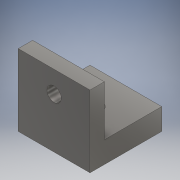
# Autodesk Inventor part: supportPoulie
Saved by Autodesk Inventor 2017 (Build 210142000, 142)
## iProperties
Created: 2017-10-26
Part Number: supportPoulie
Material: Stainless Steel
Document SubType Name: Modeling
Designer: Biscuit
Density: 8 g/cm^3
Appearance: Semi-Polished
Author: Biscuit
Autodesk Inventor part; units mm, degrees
ref_plane "YZ Plane" through (0, 0, 0) normal (1, 0, 0) x (0, 1, 0)
ref_plane "XZ Plane" through (0, 0, 0) normal (0, 1, 0) x (-1, 0, 0)
ref_plane "XY Plane" through (0, 0, 0) normal (0, 0, 1) x (1, 0, 0)
sketch "Sketch1" plane through (0, 0, 0) normal (0, 0, 1) x (1, 0, 0)
  line L0 (0, 0) -> (10, 0)
  line L1 (10, 0) -> (10, 10)
  line L2 (10, 10) -> (0, 10)
  line L3 (0, 10) -> (0, 0)
  circle A0 centre (5, 5) radius 1.5
  dimension "d0" = 10
  dimension "d1" = 10
  dimension "d8" = 3
  constraints: 8 end point, 2 parallel, 1 centre point, 1 horizontal, 1 perpendicular
  measures "d0" distance of L1.end L2.end
  measures "d1" distance of L0.end L1.end
  measures "d8" diameter of A0
extrude "Extrusion1" add sketch "Sketch1" along normal blind 3
sketch "Sketch4" plane through (0, 0, 3) normal (0, 0, 1) x (1, 0, 0)
  line L0 (10, 0) -> (10, 10) projected
  line L1 (0, 0) -> (10, 0)
  line L2 (10, 0) -> (10, 2)
  line L3 (10, 2) -> (0, 2)
  line L4 (0, 2) -> (0, 0)
  dimension "d9" = 2
  constraints: 8 end point, 2 parallel, 1 horizontal, 1 perpendicular, 1 point on line
  measures "d9" distance of L3.end L1.start
extrude "Extrusion2" add sketch "Sketch4" along normal blind 7
sketch "Sketch5" plane through (0, 0, 0) normal (0, -1, 0) x (1, 0, 0)
  circle A0 centre (5, 7) radius 1
  line L0 (10, 0) -> (10, 10) projected
  line L1 (0, 0) -> (0, 10) projected
  line L2 (0, 0) -> (10, 0) projected
  line L3 (0, 10) -> (10, 10) projected
  dimension "d12" = 10
  dimension "d13" = 10
  dimension "d14" = 7
  dimension "d15" = 5
  dimension "d16" = 2
  constraints: 1 centre point
  measures "d12" distance between parallel lines of L0 L1
  measures "d13" distance between parallel lines of L2 L3
  measures "d14" distance from line of L2 A0.centre
  measures "d15" distance from line of L0 A0.centre
  measures "d16" diameter of A0
extrude "Extrusion3" cut sketch "Sketch5" against normal through all contours A0
equation "\"d15\" = 0.5 * d12"
body "Solid1"
